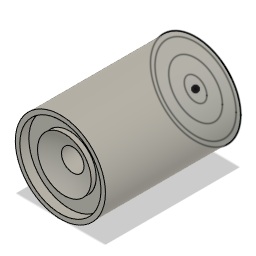
drivecup v4 (Autodesk Fusion 360 design; units mm, degrees)
Autodesk Fusion 360 part; units mm, degrees
sketch "Sketch1" plane through (0, 0, 0) normal (0, 0, 1) x (1, 0, 0)
  circle A0 centre (0, 0) radius 10
  circle A1 centre (0, 0) radius 9
  circle A2 centre (0, 0) radius 5.95
  circle A3 centre (0, 0) radius 2.5
  dimension "d1" = 20
  dimension "d2" = 18
  dimension "d3" = 11.9
  dimension "d8" = 5
  constraint coincident A0.centre A1.centre
  constraint concentric A0 A1
  constraint concentric A1 A3
  measures "d1" diameter of A0
  measures "d2" diameter of A1
  measures "d3" diameter of A2
  measures "d8" diameter of A3
extrude "Extrude1" add sketch "Sketch1" along normal blind 30 makes body 1 at (9.9503, -0.9957, 20) makes body 2 at (5.9204, -0.5924, 20)
extrude "Extrude2" add sketch "Sketch1" along normal blind 28 contours A1 bodies 1
sketch "Sketch2" plane through (0, 0, 0) normal (1, 0, 0) x (0, 0, -1)
  circle A0 centre (-30, 7.5) radius 1.5
  arc A1 (-36, -9.093) -> (-26.907, 0) centre (-36, 0) ccw
  line L0 (-1.75, 0) -> (-22.5, 0)
  line L1 (-26.907, 0) -> (-36, 0)
  line L2 (-36, 0) -> (-36, -9.093)
  dimension "d10" = 3
  dimension "d11" = 7.5
  dimension "d13" = 36
  constraint coincident A1.centre L0
  constraint coincident A1.end L0
  constraint coincident A1.centre L1.end
  constraint coincident A1 L2.end
  constraint perpendicular L1 L2
  constraint coincident A1.start L2
  measures "d10" diameter of A0
  measures "d11" vertical distance of A0.centre origin
  measures "d13" distance of origin A1.centre
revolve "Revolve1" cut sketch "Sketch2" angle 360 about axis through (0, 0, 1.75) along (0, 0, 1) contours A1 L1 L2 bodies 2
equation "d3 = d2 - ( 2 * 3.05 ) * 1 mm"
equation "d8 = stepperaxis"
equation "stepperaxis = 5 mm"
